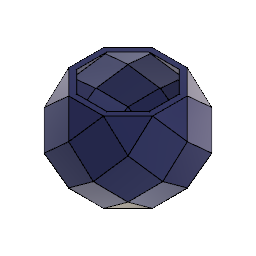
Geometric pot project (Autodesk Fusion 360 design; units mm, degrees)
Autodesk Fusion 360 part; units mm, degrees
sketch "Circumference of pot" plane through (0, 0, 0) normal (0, 0, 1) x (1, 0, 0)
  line L0 (16.5685, 40) -> (-16.5685, 40)
  line L1 (-16.5685, 40) -> (-40, 16.5685)
  line L2 (-40, 16.5685) -> (-40, -16.5685)
  line L3 (-40, -16.5685) -> (-16.5685, -40)
  line L4 (-16.5685, -40) -> (16.5685, -40)
  line L5 (16.5685, -40) -> (40, -16.5685)
  line L6 (40, -16.5685) -> (40, 16.5685)
  line L7 (40, 16.5685) -> (16.5685, 40)
  circle A0 centre (0, 0) radius 43.2957 construction
  dimension "d1" = 40
  constraint coincident A0.centre origin
  constraint horizontal L4
  constraint coincident L4.end A0
  measures "d1" distance of A0.centre L7
ref_plane "WorkPlane1" through (0, -40, 0) normal (0, -1, 0) x (1, 0, 0)
sketch "patch" plane through (0, -40, 0) normal (0, -1, 0) x (-1, 0, 0)
  line L0 (16.5685, 0) -> (-16.5685, 0) construction
  line L1 (16.5685, 0) -> (0, -15)
  line L2 (0, -15) -> (-16.5685, 0)
  line L3 (-16.5685, 0) -> (0, 12)
  line L4 (0, 12) -> (16.5685, 0)
  dimension "d4" = 15
  dimension "d5" = 12
  constraint coincident L0.start L1.start
  constraint coincident L0.end L2.end
  measures "d4" distance of L0 L1.end
  measures "d5" distance of origin L3.end
surface "SurfacePatch1" add patch profiles "patch" section 1 makes body 1
pattern_circular "C-Pattern1" count 8 over 360 about axis through (0, 0, 1.75) along (0, 0, 1) of bodies 1 makes body 2 at (24.379, -32.1895, 1) makes body 3 at (40, -5.5228, 1) makes body 4 at (32.1895, 24.379, 1) makes body 5 at (5.5228, 40, 1) makes body 6 at (-24.379, 32.1895, 1) makes body 7 at (-40, 5.5228, 1) makes body 8 at (-32.1895, -24.379, 1)
ref_plane "WorkPlane2" through (16.5685, -40, 0) normal (0.352487, -0.850978, 0.389346) x (0.92388, 0.382683, 0)
sketch "Sketch3" plane through (14.0569, -33.9364, 15.5268) normal (0.352487, -0.850978, 0.389346) x (0.92388, 0.382683, 0)
  line L0 (0, -16.857) -> (15.3073, -0.572)
  line L1 (-15.3073, -0.572) -> (0, -16.857)
  line L2 (-15.3073, -0.572) -> (0, 15.7131)
  line L3 (0, 15.7131) -> (15.3073, -0.572)
  constraint coincident L1.start L2.start
  constraint coincident L0.end L3.end
  constraint equal L2 L3
  constraint equal L0 L3
surface "SurfacePatch2" add patch profiles "Sketch3" section 1 separate body makes body 9
pattern_circular "C-Pattern2" count 8 over 360 about axis through (0, 0, 1.75) along (0, 0, 1) of bodies 9 makes body 10 at (32.1895, -13.3333, 20) makes body 11 at (32.1895, 13.3333, 20) makes body 12 at (13.3333, 32.1895, 20) makes body 13 at (-13.3333, 32.1895, 20) makes body 14 at (-32.1895, 13.3333, 20) makes body 15 at (-32.1895, -13.3333, 20) makes body 16 at (-13.3333, -32.1895, 20)
ref_plane "WorkPlane3" through (0, -40, 15) normal (0, -0.788101, 0.615545) x (1, 0, 0)
sketch "Sketch4" plane through (0, -32.1208, 25.0879) normal (0, -0.788101, 0.615545) x (1, 0, 0)
  line L0 (0, -12.8003) -> (11.7157, 6.2328)
  line L1 (-11.7157, 6.2328) -> (0, -12.8003)
  line L2 (11.7157, 6.2328) -> (-11.7157, 6.2328)
  constraint coincident L0.end L2.start
  constraint coincident L1.start L2.end
surface "SurfacePatch3" add patch profiles "Sketch4" section 1 separate body makes body 17
pattern_circular "C-Pattern3" count 8 over 360 about axis through (0, 0, 1.75) along (0, 0, 1) of bodies 17 makes body 18 at (22.7614, -22.7614, 25) makes body 19 at (32.1895, 0, 25) makes body 20 at (22.7614, 22.7614, 25) makes body 21 at (0, 32.1895, 25) makes body 22 at (-22.7614, 22.7614, 25) makes body 23 at (-32.1895, 0, 25) makes body 24 at (-22.7614, -22.7614, 25)
ref_plane "WorkPlane4" through (16.5685, -40, 0) normal (0.338356, -0.816863, -0.467172) x (0.92388, 0.382683, 0)
sketch "Sketch5" plane through (12.9525, -31.27, -17.8836) normal (0.338356, -0.816863, -0.467172) x (0.92388, 0.382683, 0)
  line L0 (0, 20.2265) -> (-15.3073, 6.6544)
  line L1 (15.3073, 6.6544) -> (0, 20.2265)
  line L2 (-15.3073, 6.6544) -> (0, -6.9177)
  line L3 (0, -6.9177) -> (15.3073, 6.6544)
  constraint coincident L0.end L2.start
  constraint coincident L1.start L3.end
  constraint equal L2 L3
  constraint equal L1 L3
surface "SurfacePatch4" add patch profiles "Sketch5" section 1 separate body makes body 25
pattern_circular "C-Pattern4" count 8 over 360 about axis through (0, 0, 1.75) along (0, 0, 1) of bodies 25 makes body 26 at (36.0948, -9.4281, -12) makes body 27 at (32.1895, 18.8562, -12) makes body 28 at (9.4281, 36.0948, -12) makes body 29 at (-9.4281, 36.0948, -12) makes body 30 at (-36.0948, 9.4281, -12) makes body 31 at (-32.1895, -18.8562, -12) makes body 32 at (-9.4281, -36.0948, -12)
ref_plane "WorkPlane5" through (0, -40, -12) normal (0, 0.715531, 0.698581) x (-1, 0, 0)
sketch "Sketch6" plane through (0, -26.4777, -25.8504) normal (0, 0.715531, 0.698581) x (-1, 0, 0)
  line L0 (11.7157, 2.5861) -> (0, 19.3569)
  line L1 (0, 19.3569) -> (-11.7157, 2.5861)
  line L2 (11.7157, 2.5861) -> (-11.7157, 2.5861)
  constraint coincident L0.start L2.start
  constraint coincident L1.end L2.end
surface "SurfacePatch5" add patch profiles "Sketch6" section 1 separate body makes body 33
pattern_circular "C-Pattern5" count 8 over 360 about axis through (0, 0, 1.75) along (0, 0, 1) of bodies 33 makes body 34 at (22.7614, -22.7614, -20) makes body 35 at (32.1895, 0, -20) makes body 36 at (22.7614, 22.7614, -20) makes body 37 at (0, 32.1895, -20) makes body 38 at (-22.7614, 22.7614, -20) makes body 39 at (-32.1895, 0, -20) makes body 40 at (-22.7614, -22.7614, -20)
stitch "SurfaceStitch1" surfaces 36 16 5 20 17 38 7 9 39 22 24 26 35 6 27 21 33 12 15 10 4 34 13 32 29 19 14 40 28 11 31 3 37 1 25 2 18 23 8 30 tolerance 0.1 makes body 41
surface "SurfacePatch6" add patch along 8 edges at (0, -28.2843, 30) (-20, -20, 30) (-28.2843, 0, 30) (-20, 20, 30) (0, 28.2843, 30) (20, 20, 30) (28.2843, 0, 30) (20, -20, 30) separate body on bodies 41 makes body 42
surface "SurfacePatch7" add patch along 8 edges at (-20, 20, -24) (-28.2843, 0, -24) (-20, -20, -24) (0, -28.2843, -24) (20, -20, -24) (28.2843, 0, -24) (20, 20, -24) (0, 28.2843, -24) separate body on bodies 41 makes body 43
stitch "SurfaceStitch2" surfaces 41 42 43 tolerance 0.1 makes body 44
shell "Shell1" thickness 3 removed faces 1 at (-1.6176, -3.9052, 30) on bodies 44
sketch "Sketch7" plane through (0, 0, 0) normal (0, 0, 1) x (1, 0, 0)
  circle A0 centre (0, 0) radius 5
  dimension "d19" = 10
  constraint coincident A0.centre origin
  measures "d19" diameter of A0
extrude "Extrude1" cut sketch "Sketch7" against normal blind 230 bodies 44
named bodies: "Flower pot"
